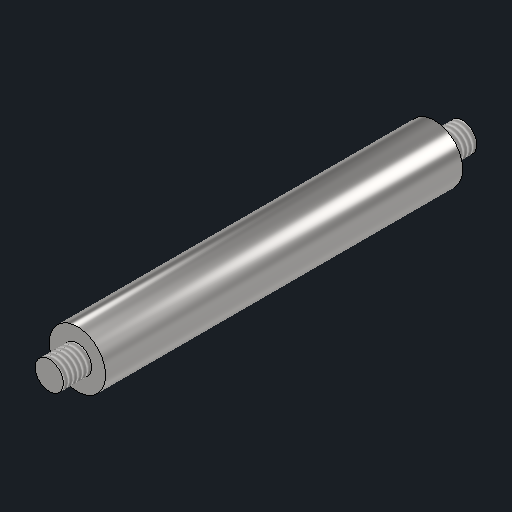
# Autodesk Inventor part: Shaft
Saved by Autodesk Inventor 2027.1 (Build 311270010, 270A)
## iProperties
Created: 2025-06-19
Part Number: Shaft
Material: Stainless Steel
Document SubType Name: Modeling
Designer: kuzmin
Density: 8 g/cm^3
Appearance: Semi-Polished
Author: kuzmin
Autodesk Inventor part; units mm, degrees
ref_plane "YZ Plane" through (0, 0, 0) normal (1, 0, 0) x (0, 1, 0)
ref_plane "XZ Plane" through (0, 0, 0) normal (0, 1, 0) x (-1, 0, 0)
ref_plane "XY Plane" through (0, 0, 0) normal (0, 0, 1) x (1, 0, 0)
sketch "Sketch1" plane through (0, 0, 0) normal (0, 1, 0) x (-1, 0, 0)
  line L0 (0, -22) -> (0, 22)
  line L1 (0, 22) -> (1.5, 22)
  line L2 (1.5, 22) -> (1.5, 19)
  line L3 (1.5, 19) -> (3, 19)
  line L4 (3, 19) -> (3, -19)
  line L5 (3, -19) -> (1.5, -19)
  line L6 (1.5, -19) -> (1.5, -22)
  line L7 (1.5, -22) -> (0, -22)
  point P0 (0, 0)
  point P1 (0, 0)
  point P2 (3, 0)
  dimension "d1" = 6
  dimension "d2" = 3
  dimension "d3" = 3
  dimension "d4" = 44
  constraints: 16 end point, 6 perpendicular, 2 midpoint, 1 coincident, 1 horizontal, 1 horizontal alignment, 1 vertical, 1 vertical alignment
  measures "d1" diameter of L4 L0
  measures "d2" diameter of L2 L0
  measures "d3" distance of L1.end L2.end
  measures "d4" distance of L0.start L0.end
revolve "Revolution1" add sketch "Sketch1" angle 360 about axis through (0, 0, -22) along (0, 0, 1)
thread "Thread1" size "M3x0.5" class "6g" standard "ANSI Metric M Profile" full length
thread "Thread2" size "M3x0.5" class "6g" standard "ANSI Metric M Profile" full length
equation "\"d4\" = L"
equation "\"L\" = 44"
body "Solid1"
